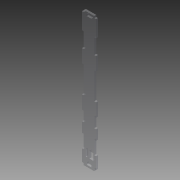
# Autodesk Inventor part: Left_wall
Saved by Autodesk Inventor 2015 (Build 190159000, 159)
## iProperties
Created: 2015-06-19
Part Number: Left_wall
Material: Generic
Document SubType Name: Modeling
Designer: Openlab
Density: 1 g/cm^3
Appearance: Polycarbonate - Clear
Author: Openlab
Autodesk Inventor part; units mm, degrees
ref_plane "YZ Plane" through (0, 0, 0) normal (1, 0, 0) x (0, 1, 0)
ref_plane "XZ Plane" through (0, 0, 0) normal (0, 1, 0) x (-1, 0, 0)
ref_plane "XY Plane" through (0, 0, 0) normal (0, 0, 1) x (1, 0, 0)
sketch "Sketch1" plane through (0, 0, 0) normal (0, 1, 0) x (-1, 0, 0)
  line L0 (21, -25) -> (18.25, -25)
  line L1 (21, -48) -> (18.25, -48)
  line L2 (21, -143) -> (18.25, -143)
  line L3 (21, -68) -> (18.25, -68)
  line L4 (21, -128) -> (18.25, -128)
  line L5 (21, -108) -> (18.25, -108)
  line L6 (2.75, -68) -> (0, -68)
  line L7 (2.75, -108) -> (0, -108)
  line L8 (2.75, -128) -> (0, -128)
  line L9 (2.75, -143) -> (0, -143)
  line L10 (2.75, -48) -> (0, -48)
  line L11 (2.75, -25) -> (0, -25)
  line L12 (21, -158) -> (21, -143)
  line L13 (21, -128) -> (21, -108)
  line L14 (21, -68) -> (21, -48)
  line L15 (21, -25) -> (21, 0)
  line L16 (0, -158) -> (0, -143)
  line L17 (0, -128) -> (0, -108)
  line L18 (0, -68) -> (0, -48)
  line L19 (0, -25) -> (0, 0)
  line L20 (18.25, -143) -> (18.25, -128)
  line L21 (18.25, -108) -> (18.25, -68)
  line L22 (18.25, -48) -> (18.25, -25)
  line L23 (2.75, -143) -> (2.75, -128)
  line L24 (2.75, -108) -> (2.75, -68)
  line L25 (2.75, -48) -> (2.75, -25)
  line L26 (21, -68) -> (21, -48) construction
  line L27 (2.75, -178) -> (2.75, -158)
  line L28 (21, -158) -> (18.25, -158)
  line L29 (2.75, -158) -> (0, -158)
  line L30 (18.25, -158) -> (18.25, -178)
  line L31 (18.25, -178) -> (21, -178)
  line L32 (21, -178) -> (21, -196)
  line L33 (0, -196) -> (0, -178)
  line L34 (0, -178) -> (2.75, -178)
  line L35 (15.25, -176) -> (13.45, -176)
  line L36 (13.45, -176) -> (13.45, -186)
  line L37 (13.45, -186) -> (15.25, -186)
  line L38 (15.25, -186) -> (15.25, -176)
  line L39 (18.25, -196) -> (18.25, -198.75)
  line L40 (18.25, -198.75) -> (2.75, -198.75)
  line L41 (2.75, -198.75) -> (2.75, -196)
  line L42 (21, -196) -> (18.25, -196)
  line L43 (2.75, -196) -> (0, -196)
  line L44 (18.25, 0) -> (18.25, 2.75)
  line L45 (18.25, 2.75) -> (2.75, 2.75)
  line L46 (2.75, 2.75) -> (2.75, 0)
  line L47 (21, 0) -> (18.25, 0)
  line L48 (2.75, 0) -> (0, 0)
  line L49 (14, -193) -> (7, -193)
  line L50 (7, -193) -> (7, -196)
  line L51 (7, -196) -> (14, -196)
  line L52 (14, -196) -> (14, -193)
  line L53 (14, 0) -> (7, 0)
  line L54 (7, 0) -> (7, -3)
  line L55 (7, -3) -> (14, -3)
  line L56 (14, -3) -> (14, 0)
  line L57 (10.5, -82) -> (10.5, -115) construction
  line L58 (9.95, -176) -> (3.95, -176)
  line L59 (3.95, -176) -> (3.95, -186)
  line L60 (3.95, -186) -> (9.95, -186)
  line L61 (9.95, -186) -> (9.95, -176)
  dimension "d7" = 23
  dimension "d8" = 20
  dimension "d9" = 40
  dimension "d10" = 20
  dimension "d11" = 15
  dimension "d28" = 15.5
  dimension "d31" = 2.75
  dimension "d38" = 15
  dimension "d39" = 20
  dimension "d40" = 18
  dimension "d43" = 1.8
  dimension "d45" = 10
  dimension "d46" = 3
  dimension "d47" = 10
  dimension "d48" = 25
  dimension "d49" = 3
  dimension "d50" = 7
  dimension "d51" = 3.5
  dimension "d52" = 6
  constraints: 125 end point, 38 collinear, 17 perpendicular, 14 parallel, 6 vertical, 5 equal length, 4 horizontal, 2 point on line, 3 other
  measures "d7" distance between parallel lines of L1 L0
  measures "d8" distance between parallel lines of L3 L1
  measures "d9" distance between parallel lines of L5 L3
  measures "d10" distance between parallel lines of L4 L5
  measures "d11" distance between parallel lines of L2 L4
  measures "d28" distance between parallel lines of L23 L20
  measures "d31" distance between parallel lines of L22 L15
  measures "d38" distance of L12.start L2.start
  measures "d39" distance of L28.end L30.end
  measures "d40" distance of L31.end L32.end
  measures "d43" distance of L35.start L35.end
  measures "d45" distance of L37.end L35.start
  measures "d46" distance between parallel lines of L38 L30
  measures "d47" distance between parallel lines of L42 L37
  measures "d48" distance between parallel lines of L0 L47
  measures "d49" distance of L53.end L54.end
  measures "d50" distance of L54.end L55.end
  measures "d51" distance between parallel lines of L36 L61
  measures "d52" distance of L58.start L58.end
extrude "Extrusion3" add sketch "Sketch1" along normal blind 3
body "Solid3"
